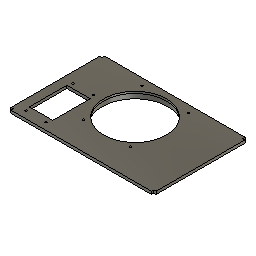
printplate holder bottom v3 (Autodesk Fusion 360 design; units mm, degrees)
Autodesk Fusion 360 part; units mm, degrees
sketch "Skizze1" plane through (0, 0, 0) normal (0, 0, 1) x (1, 0, 0)
  line L0 (0, 0) -> (240, 0)
  line L1 (240, 0) -> (240, 240)
  line L2 (240, 240) -> (0, 240)
  line L3 (0, 240) -> (0, 0)
  dimension "d1" = 240
  dimension "d2" = 240
  constraint horizontal L0
  constraint vertical L1
  constraint horizontal L2
  constraint vertical L3
  constraint coincident L0.start L3.end
  measures "d1" distance of L0.start L0.end
  measures "d2" distance of L0.start L2.end
extrude "Extrusion1" add sketch "Skizze1" along normal blind 6
sketch "Skizze2" plane through (0, 0, 6) normal (0, 0, 1) x (-1, 0, 0)
  line L0 (0, -240) -> (0, 0)
  line L1 (0, 0) -> (-240, 0)
  line L2 (-240, 0) -> (-240, -240)
  line L3 (-240, -240) -> (0, -240)
  circle A0 centre (-150, -160) radius 70
  dimension "d6" = 140
  measures "d6" diameter of A0
extrude "Extrusion2" cut sketch "Skizze2" against normal blind 2 contours A0
sketch "Skizze3" plane through (0, 0, 4) normal (0, 0, 1) x (-1, 0, 0)
  circle A0 centre (-150, -160) radius 70
  circle A1 centre (-150, -160) radius 67
  dimension "d9" = 134
  constraint concentric A0 A1
  measures "d9" diameter of A1
extrude "Extrusion3" cut sketch "Skizze3" against normal blind 35 contours A1
extrude "Extrusion4" add 1 faces at (208.7542, 124.1511, 4) along direction (0, 0, 1) blind 2
sketch "Skizze4" plane through (0, 0, 0) normal (0, 0, -1) x (1, 0, 0)
  circle A0 centre (150, -160) radius 67
  line L0 (0, 0) -> (0, -240)
  line L1 (0, -240) -> (240, -240)
  line L2 (240, -240) -> (240, 0)
  line L3 (240, 0) -> (0, 0)
  circle A1 centre (150, -160) radius 70
  dimension "d14" = 140
  constraint concentric A0 A1
  measures "d14" diameter of A1
extrude "Extrusion5" cut sketch "Skizze4" against normal blind 2 contours A1
extrude "Extrusion6" cut 1 faces at (80, 0, 2) along direction (0, 1, 0) blind 40
sketch "Skizze5" plane through (0, 0, 0) normal (0, 0, -1) x (1, 0, 0)
  line L0 (240, -40) -> (0, -40)
  line L1 (0, -40) -> (0, -240)
  line L2 (0, -240) -> (240, -240)
  line L3 (240, -240) -> (240, -40)
  circle A0 centre (150, -160) radius 70
  circle A1 centre (150, -160) radius 70
  circle A2 centre (150, -160) radius 72
  dimension "d19" = 144
  constraint concentric A0 A1
  constraint concentric A1 A2
  measures "d19" diameter of A2
extrude "Extrusion7" add sketch "Skizze5" along normal blind 10 contours A2
extrude "Extrusion8" add 1 faces at (240, 106.6667, 4) along direction (1, 0, 0) blind 70
sketch "Skizze6" plane through (0, 0, 0) normal (0, 0, -1) x (1, 0, 0)
  circle A0 centre (150, -160) radius 72
  line L0 (310, -40) -> (0, -40)
  line L1 (0, -40) -> (0, -240)
  line L2 (0, -240) -> (310, -240)
  line L3 (310, -240) -> (310, -40)
  line L4 (0, -40) -> (5, -40)
  line L5 (5, -40) -> (5, -45)
  line L6 (5, -45) -> (0, -45)
  line L7 (0, -45) -> (0, -40)
  line L8 (0, -240) -> (5, -240)
  line L9 (5, -240) -> (5, -235)
  line L10 (5, -235) -> (0, -235)
  line L11 (0, -235) -> (0, -240)
  line L12 (310, -240) -> (305, -240)
  line L13 (305, -240) -> (305, -235)
  line L14 (305, -235) -> (310, -235)
  line L15 (310, -235) -> (310, -240)
  line L16 (310, -40) -> (305, -40)
  line L17 (305, -40) -> (305, -45)
  line L18 (305, -45) -> (310, -45)
  line L19 (310, -45) -> (310, -40)
  dimension "d24" = 5
  dimension "d25" = 5
  constraint horizontal L4
  constraint vertical L5
  constraint horizontal L6
  constraint vertical L7
  constraint coincident L0.end L1.start
  constraint horizontal L8
  constraint vertical L9
  constraint horizontal L10
  constraint vertical L11
  constraint coincident L1.end L2.start
  constraint horizontal L12
  constraint vertical L13
  constraint horizontal L14
  constraint vertical L15
  constraint coincident L2.end L3.start
  constraint horizontal L16
  constraint vertical L17
  constraint horizontal L18
  constraint vertical L19
  constraint coincident L0.start L3.end
  measures "d24" distance of L0.end L4.end
  measures "d25" distance of L0.end L6.end
extrude "Extrusion9" cut sketch "Skizze6" against normal blind 20 contours L0 L3 L16 L17 L18 L19 | L0 L1 L4 L5 L6 L7 | L2 L3 L12 L13 L14 L15 | L1 L2 L8 L9 L10 L11
sketch "Skizze7" plane through (0, 0, 0) normal (0, 0, -1) x (1, 0, 0)
  circle A0 centre (150, -160) radius 72
  line L0 (305, -240) -> (305, -235)
  line L1 (305, -235) -> (310, -235)
  line L2 (310, -235) -> (310, -45)
  line L3 (310, -45) -> (305, -45)
  line L4 (305, -45) -> (305, -40)
  line L5 (305, -40) -> (5, -40)
  line L6 (5, -40) -> (5, -45)
  line L7 (5, -45) -> (0, -45)
  line L8 (0, -45) -> (0, -235)
  line L9 (0, -235) -> (5, -235)
  line L10 (5, -235) -> (5, -240)
  line L11 (5, -240) -> (305, -240)
  line L12 (18.5416, -65.8113) -> (68.5416, -65.8113)
  line L13 (68.5416, -65.8113) -> (68.5416, -145.8113)
  line L14 (68.5416, -145.8113) -> (18.5416, -145.8113)
  line L15 (18.5416, -145.8113) -> (18.5416, -65.8113)
  circle A1 centre (64.5928, -155.8111) radius 2
  circle A2 centre (22.0928, -155.8111) radius 2
  circle A3 centre (64.5928, -55.1368) radius 2
  circle A4 centre (22.0928, -55.1368) radius 2
  dimension "d28" = 80
  dimension "d29" = 42.5
  dimension "d30" = 4
  dimension "d31" = 4
  dimension "d32" = 4
  dimension "d33" = 4
  constraint horizontal L12
  constraint vertical L13
  constraint horizontal L14
  constraint vertical L15
  measures "d28" distance of L12.start L14.end
  measures "d29" distance of A1.centre A2.centre
  measures "d30" diameter of A1
  measures "d31" diameter of A2
  measures "d32" diameter of A3
  measures "d33" diameter of A4
extrude "Extrusion10" cut sketch "Skizze7" against normal blind 90 contours L12 L13 L14 L15 | A1 | A2 | A3 | A4
sketch "Skizze8" plane through (0, 0, 6) normal (0, 0, 1) x (-1, 0, 0)
  line L0 (-68.5416, -145.8113) -> (-68.5416, -65.8113)
  line L1 (-68.5416, -65.8113) -> (-18.5416, -65.8113)
  line L2 (-18.5416, -65.8113) -> (-18.5416, -145.8113)
  line L3 (-18.5416, -145.8113) -> (-68.5416, -145.8113)
  circle A0 centre (-64.5928, -155.8111) radius 2
  circle A1 centre (-64.5928, -55.1368) radius 2
  circle A2 centre (-22.0928, -155.8111) radius 2
  circle A3 centre (-22.0928, -55.1368) radius 2
  circle A4 centre (-150, -160) radius 67
  line L4 (-310, -235) -> (-305, -235)
  line L5 (-305, -235) -> (-305, -240)
  line L6 (-305, -240) -> (-5, -240)
  line L7 (-5, -240) -> (-5, -235)
  line L8 (-5, -235) -> (0, -235)
  line L9 (0, -235) -> (0, -45)
  line L10 (0, -45) -> (-5, -45)
  line L11 (-5, -45) -> (-5, -40)
  line L12 (-5, -40) -> (-305, -40)
  line L13 (-305, -40) -> (-305, -45)
  line L14 (-305, -45) -> (-310, -45)
  line L15 (-310, -45) -> (-310, -235)
  circle A5 centre (-100, -225) radius 2
  circle A6 centre (-200, -225) radius 2
  circle A7 centre (-200, -100) radius 2
  circle A8 centre (-100, -100) radius 2
  dimension "d36" = 4
  dimension "d37" = 4
  dimension "d38" = 4
  dimension "d39" = 4
  measures "d36" diameter of A5
  measures "d37" diameter of A6
  measures "d38" diameter of A7
  measures "d39" diameter of A8
extrude "Extrusion11" cut sketch "Skizze8" against normal blind 3 contours A5 | A6 | A7 | A8
